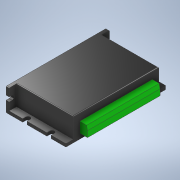
# Autodesk Inventor part: CL57T_Stepper_Driver
Saved by Autodesk Inventor 2020 (Build 240168000, 168)
## iProperties
Created: 2019-11-19
Part Number: CL57T_Stepper_Driver
Material: Generic
Document SubType Name: Modeling
Designer: kylew
Density: 1 g/cm^3
Appearance: Default
Author: kylew
Autodesk Inventor part; units mm, degrees
ref_plane "YZ Plane" through (0, 0, 0) normal (1, 0, 0) x (0, 1, 0)
ref_plane "XZ Plane" through (0, 0, 0) normal (0, 1, 0) x (-1, 0, 0)
ref_plane "XY Plane" through (0, 0, 0) normal (0, 0, 1) x (1, 0, 0)
sketch "Sketch1" plane through (0, 0, 0) normal (0, 1, 0) x (-1, 0, 0)
  line L0 (34.6, 58) -> (-34.6, 58)
  line L1 (-34.6, 58) -> (-34.6, -58)
  line L2 (-34.6, -58) -> (34.6, -58)
  line L3 (34.6, -58) -> (34.6, 58)
  line L4 (34.6, 58) -> (-34.6, -58) construction
  line L5 (-34.6, 58) -> (34.6, -58) construction
  point P0 (0, 0)
  dimension "d0" = 69.2
  dimension "d1" = 116
  constraints: 12 end point, 2 midpoint, 2 parallel, 1 horizontal, 1 perpendicular
  measures "d0" distance of L2.end L1.end
  measures "d1" distance of L1.end L0.end
extrude "Extrusion1" add sketch "Sketch1" along normal blind 3.5
sketch "Sketch2" plane through (0, 3.5, 0) normal (0, 1, 0) x (1, 0, 0)
  line L0 (-34.6, 49.5) -> (34.6, 49.5)
  line L1 (34.6, 49.5) -> (34.6, -49.5)
  line L2 (34.6, -49.5) -> (-34.6, -49.5)
  line L3 (-34.6, -49.5) -> (-34.6, 49.5)
  line L4 (-34.6, 49.5) -> (34.6, -49.5) construction
  line L5 (34.6, 49.5) -> (-34.6, -49.5) construction
  line L6 (-34.6, 49.5) -> (-31.1, 49.5)
  line L7 (-31.1, 49.5) -> (-31.1, 58)
  line L8 (-31.1, 58) -> (-34.6, 58)
  line L9 (-34.6, 58) -> (-34.6, 49.5)
  line L10 (-34.6, -49.5) -> (-31.1, -49.5)
  line L11 (-31.1, -49.5) -> (-31.1, -58)
  line L12 (-31.1, -58) -> (-34.6, -58)
  line L13 (-34.6, -58) -> (-34.6, -49.5)
  point P0 (0, 0)
  dimension "d4" = 69.2
  dimension "d5" = 99
  dimension "d6" = 3.5
  dimension "d7" = 8.5
  dimension "d8" = 3.5
  dimension "d9" = 8.5
  constraints: 28 end point, 6 parallel, 3 horizontal, 3 perpendicular, 2 midpoint
  measures "d4" distance of L1.end L2.end
  measures "d5" distance of L0.end L1.end
  measures "d6" distance of L8.end L7.end
  measures "d7" distance of L7.end L6.end
  measures "d8" distance of L11.end L12.end
  measures "d9" distance of L10.end L11.end
extrude "Extrusion2" add sketch "Sketch2" along normal blind 23
sketch "Sketch3" plane through (34.6, 0, 58) normal (1, 0, 0) x (0, 0, -1)
  line L0 (58, 0) -> (58, 55) construction
  line L1 (58, 0) -> (113, 0) construction
  line L2 (16, 18) -> (100, 18)
  line L3 (100, 18) -> (100, 6)
  line L4 (100, 6) -> (16, 6)
  line L5 (16, 6) -> (16, 18)
  line L6 (16, 18) -> (100, 6) construction
  line L7 (100, 18) -> (16, 6) construction
  point P0 (58, 12)
  dimension "d12" = 55
  dimension "d13" = 90
  dimension "d14" = 84
  dimension "d15" = 12
  dimension "d16" = 12
  constraints: 16 end point, 2 horizontal, 2 midpoint, 2 parallel, 2 perpendicular, 1 point on line, 1 vertical
  measures "d12" distance of L0.start L0.end
  measures "d13" angle of L1 L0
  measures "d14" distance of L3.end L4.end
  measures "d15" distance of L2.end L3.end
  measures "d16" distance from line of L1 point (58, 12)
extrude "Extrusion3" add sketch "Sketch3" along normal blind 9
chamfer "Chamfer1" distance 5 distance2 1 1 edges at (43.6, 18, 0) measured on face at (43.6, 14, 14)
sketch "Sketch5" plane through (-31.1, 3.5, -49.5) normal (1, 0, 0) x (0, 0, -1)
  line L0 (5, 11.5) -> (10, 11.5) construction
  line L1 (5, 9) -> (10, 9)
  line L2 (10, 14) -> (5, 14)
  arc A0 (5, 14) -> (5, 9) centre (5, 11.5) ccw
  arc A1 (10, 9) -> (10, 14) centre (10, 11.5) ccw
  line L3 (5, 11.5) -> (10, 11.5) construction
  line L4 (-107.5, -3.5) -> (8.5, -3.5) projected
  line L5 (8.5, 0) -> (8.5, 23) projected
  point P0 (-49.5, -3.5)
  point P1 (7.5, 11.5)
  point P2 (8.5, 9)
  point P3 (8.5, 14)
  dimension "d38" = 5
  dimension "d39" = 0
  dimension "d40" = 5
  dimension "d41" = 15
  dimension "d42" = 3.5
  constraints: 10 end point, 4 point on circle, 4 tangent, 2 centre point, 2 horizontal, 1 collinear, 1 midpoint, 1 parallel
  measures "d38" distance of L0.start L0.end
  measures "d39" distance between parallel lines of L0 L3
  measures "d40" diameter of A1
  measures "d41" distance from line of L4 point (7.5, 11.5)
  measures "d42" distance from line of L5 L0.start
extrude "Extrusion5" cut sketch "Sketch5" against normal blind 9 contours A0 L2 L5 L1
sketch "Sketch4" plane through (0, 3.5, 0) normal (0, 1, 0) x (1, 0, 0)
  circle A0 centre (15.1, 54.5) radius 2.5
  circle A1 centre (-12.9, 54.5) radius 2.5
  line L0 (34.6, 49.5) -> (34.6, 58) projected
  line L1 (34.6, 58) -> (-31.1, 58) projected
  line L2 (15.1, 54.5) -> (15.1, 58) construction
  line L3 (34.6, 58) -> (-34.6, 58) projected
  line L4 (17.6, 54.5) -> (17.6, 58)
  line L5 (12.6, 58) -> (12.6, 54.5)
  arc A2 (12.6, 54.5) -> (17.6, 54.5) centre (15.1, 54.5) ccw
  arc A3 (17.6, 58) -> (12.6, 58) centre (15.1, 58) ccw
  line L6 (15.1, 54.5) -> (18.6, 54.5) construction
  line L7 (-12.9, 54.5) -> (-12.9, 58) construction
  line L8 (-10.4, 54.5) -> (-10.4, 58)
  line L9 (-15.4, 58) -> (-15.4, 54.5)
  arc A4 (-15.4, 54.5) -> (-10.4, 54.5) centre (-12.9, 54.5) ccw
  arc A5 (-10.4, 58) -> (-15.4, 58) centre (-12.9, 58) ccw
  line L10 (-12.9, 54.5) -> (-9.4, 54.5) construction
  point P0 (0, 0)
  point P1 (15.1, 56.25)
  point P2 (-12.9, 56.25)
  point P3 (17.6, 54.5)
  dimension "d22" = 5
  dimension "d23" = 5
  dimension "d24" = 19.5
  dimension "d25" = 28
  dimension "d26" = 3.5
  dimension "d27" = 3.5
  dimension "d28" = 90
  dimension "d29" = 5
  dimension "d30" = 3.5
  dimension "d31" = 90
  dimension "d32" = 5
  constraints: 20 end point, 8 point on circle, 8 tangent, 6 centre point, 3 parallel, 2 horizontal, 2 midpoint, 2 perpendicular, 1 point on line
  measures "d22" diameter of A0
  measures "d23" diameter of A1
  measures "d24" distance from line of L0 L2.start
  measures "d25" distance of L7.start L2.start
  measures "d26" distance from line of L1 L7.start
  measures "d27" distance from line of L1 L2.start
  measures "d28" angle of L6 L2
  measures "d29" diameter of A3
  measures "d30" distance of L7.start L7.end
  measures "d31" angle of L10 L7
  measures "d32" diameter of A5
extrude "Extrusion4" cut sketch "Sketch4" against normal blind 9 contours A0 | L8 A1 L9 L1 | A0 L5 L1 L4 | A1
mirror "Mirror1" about plane through (0, 0, 0) normal (0, 0, 1) of "Extrusion4", "Extrusion5"
fillet "Fillet1" radius 1 8 edges at (34.6, 26.5, 0) (1.75, 26.5, 49.5) (1.75, 26.5, -49.5) (-32.85, 26.5, -58) (34.6, 1.75, -58) (34.6, 1.75, 58) (-34.6, 0, 0) (-32.85, 26.5, 58)
sketch "Sketch6" plane through (34.6, 3.5, -49.5) normal (0, 0, -1) x (-1, 0, 0)
  line L0 (34.6, -3.5) -> (34.6, 46.5) construction
  line L1 (34.6, -3.5) -> (84.6, -3.5) construction
  line L2 (47.1, 16) -> (22.1, 16)
  line L3 (22.1, 16) -> (22.1, 6)
  line L4 (22.1, 6) -> (47.1, 6)
  line L5 (47.1, 6) -> (47.1, 16)
  line L6 (47.1, 16) -> (22.1, 6) construction
  line L7 (22.1, 16) -> (47.1, 6) construction
  point P0 (34.6, 11)
  dimension "d46" = 50
  dimension "d47" = 90
  dimension "d48" = 25
  dimension "d49" = 10
  dimension "d50" = 14.5
  constraints: 16 end point, 2 horizontal, 2 midpoint, 2 parallel, 2 perpendicular, 1 point on line, 1 vertical
  measures "d46" distance of L0.start L0.end
  measures "d47" angle of L1 L0
  measures "d48" distance of L4.end L3.end
  measures "d49" distance of L3.end L2.end
  measures "d50" distance from line of L1 point (34.6, 11)
extrude "Extrusion6" cut sketch "Sketch6" against normal blind 1.5
body "Solid1"
